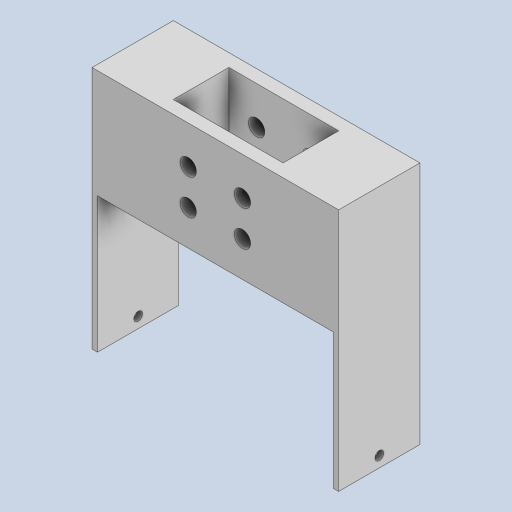
# Autodesk Inventor part: frame_arm
Saved by Autodesk Inventor 2023 (Build 270158000, 158)
## iProperties
Created: 2024-09-13
Part Number: frame_arm
Material: Generic
Document SubType Name: Modeling
Designer: kiyo
Density: 1 g/cm^3
Appearance: Default
Author: kiyo
Autodesk Inventor part; units mm, degrees
ref_plane "YZ Plane" through (0, 0, 0) normal (1, 0, 0) x (0, 1, 0)
ref_plane "XZ Plane" through (0, 0, 0) normal (0, 1, 0) x (-1, 0, 0)
ref_plane "XY Plane" through (0, 0, 0) normal (0, 0, 1) x (1, 0, 0)
sketch "スケッチ1" plane through (0, 0, 0) normal (0, 0, 1) x (1, 0, 0)
  line L0 (15, -45.5) -> (-15, -45.5)
  line L1 (-15, -45.5) -> (-15, 45.5)
  line L2 (-15, 45.5) -> (15, 45.5)
  line L3 (15, 45.5) -> (15, -45.5)
  line L4 (15, -45.5) -> (-15, 45.5) construction
  line L5 (-15, -45.5) -> (15, 45.5) construction
  line L6 (-10.25, -20.25) -> (-10.25, 20.25)
  line L7 (-10.25, 20.25) -> (10.25, 20.25)
  line L8 (10.25, 20.25) -> (10.25, -20.25)
  line L9 (10.25, -20.25) -> (-10.25, -20.25)
  line L10 (-10.25, -20.25) -> (10.25, 20.25) construction
  line L11 (-10.25, 20.25) -> (10.25, -20.25) construction
  point P0 (0, 0)
  dimension "d0" = 30
  dimension "d1" = 91
  dimension "d4" = 40.5
  dimension "d5" = 20.5
  constraints: 24 end point, 4 midpoint, 4 parallel, 2 perpendicular, 1 horizontal, 1 vertical
  measures "d0" distance of L0.start L0.end
  measures "d1" distance of L0.end L1.end
  measures "d4" distance of L6.start L6.end
  measures "d5" distance of L6.end L7.end
extrude "押し出し1" add sketch "スケッチ1" along normal blind 40
sketch "スケッチ2" plane through (0, 0, 0) normal (0, 0, -1) x (-1, 0, 0)
  line L0 (-15, -45.5) -> (-15, 45.5) projected
  line L1 (15, 45.5) -> (15, -45.5) projected
  line L2 (-15, -45.5) -> (15, -45.5)
  line L3 (15, -45.5) -> (15, -43.5)
  line L4 (15, -43.5) -> (-15, -43.5)
  line L5 (-15, -43.5) -> (-15, -45.5)
  line L6 (-15, 45.5) -> (15, 45.5) projected
  line L7 (-15, 45.5) -> (15, 45.5)
  line L8 (15, 45.5) -> (15, 43.5)
  line L9 (15, 43.5) -> (-15, 43.5)
  line L10 (-15, 43.5) -> (-15, 45.5)
  point P0 (0, 0)
  point P1 (-15, 43.5)
  dimension "d6" = 2
  dimension "d7" = 2
  constraints: 16 end point, 4 parallel, 2 horizontal, 2 perpendicular, 2 point on line
  measures "d6" distance between parallel lines of L2 L4
  measures "d7" distance between parallel lines of L6 L9
extrude "押し出し2" add sketch "スケッチ2" along normal blind 50 contours L0 L4 L1 L2 | L0 L6 L1 L9
sketch "スケッチ3" plane through (-15, 45.5, 40) normal (0, 1, 0) x (1, 0, 0)
  line L0 (0, 90) -> (30, 90) projected
  line L1 (30, 0) -> (30, 90) projected
  point P0 (15, 40)
  point P1 (15, 86)
  dimension "d10" = 4
  dimension "d11" = 15
  measures "d10" distance from line of L0 point (15, 86)
  measures "d11" distance from line of L1 point (15, 86)
hole "穴1" at (0, 45.5, -46) direction (0, -1, 0) diameter 3.2 depth 91
sketch "スケッチ4" plane through (15, -45.5, 40) normal (1, 0, 0) x (0, 0, -1)
  circle A0 centre (27, 55.5) radius 3
  line L0 (0, 0) -> (0, 91) projected
  line L1 (40, 2) -> (40, 89) projected
  line L2 (0, 91) -> (90, 91) projected
  circle A1 centre (14, 55.5) radius 3
  circle A2 centre (27, 35.5) radius 3
  circle A3 centre (14, 35.5) radius 3
  point P0 (40, 45.5)
  point P1 (0, 45.5)
  dimension "d19" = 10
  dimension "d20" = 13
  dimension "d23" = 13
  dimension "d26" = 20
  dimension "d29" = 6
  constraints: 4 centre point, 1 horizontal, 1 midpoint, 1 vertical, 6 other
  measures "d19" vertical distance of point (0, 45.5) A0.centre
  measures "d20" distance from line of L1 A0.centre
  measures "d23" distance of A0.centre A1.centre
  measures "d26" distance of A0.centre A2.centre
  measures "d29" diameter of A0
extrude "押し出し3" cut sketch "スケッチ4" against normal up to surface (30 mm away)
